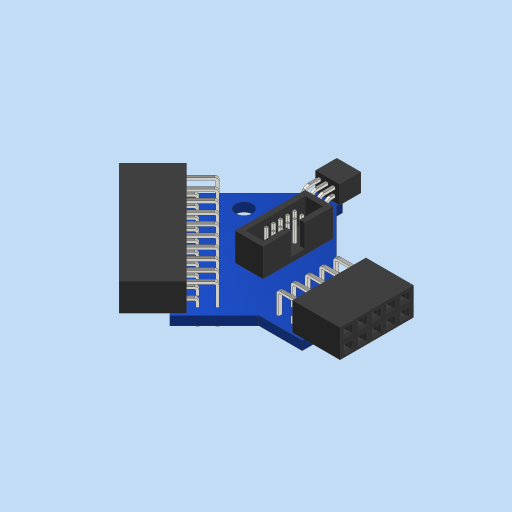
# Autodesk Inventor part: Atmel-ICE_adapter
Saved by Autodesk Inventor 2024 (Build 280153000, 153)
## iProperties
Created: 2025-05-11
Part Number: Atmel-ICE_adapter
Material: Generic
Document SubType Name: Modeling
Designer: XxPan
Density: 1 g/cm^3
Appearance: Default
Author: XxPan
Autodesk Inventor part; units mm, degrees
sketch "Sketch1" plane through (0, 0, 0) normal (0, 1, 0) x (-1, 0, 0)
  line L0 (0, 0) -> (0, -13.9)
  line L1 (0, -13.9) -> (7.7796, -13.9)
  line L2 (7.7796, -13.9) -> (17.78, -23.9005)
  line L3 (17.78, -23.9005) -> (17.78, -25.03)
  line L4 (17.78, -25.03) -> (21.78, -25.03)
  line L5 (21.78, -25.03) -> (21.78, -23.9005)
  line L6 (21.78, -23.9005) -> (34.7, -10.9805)
  line L7 (34.7, -10.9805) -> (26.2854, -2.5659)
  line L8 (26.2854, -2.5659) -> (30.8109, 1.9595)
  line L9 (30.8109, 1.9595) -> (28.6896, 4.0809)
  line L10 (28.6896, 4.0809) -> (24.1641, -0.4446)
  line L11 (24.1641, -0.4446) -> (15.7495, 7.97)
  line L12 (15.7495, 7.97) -> (7.7796, 0)
  line L13 (7.7796, 0) -> (0, 0)
  dimension "d0" = 135
  dimension "d1" = 135
  dimension "d2" = 21.1
  dimension "d3" = 13.9
  dimension "d4" = 26.8
  dimension "d5" = 11.9
  dimension "d7" = 11.9
  dimension "d8" = 6.4
  dimension "d9" = 33
  dimension "d10" = 34.7
  dimension "d11" = 4
  constraints: 28 end point, 8 perpendicular, 2 point on line, 1 horizontal alignment, 1 parallel, 1 vertical, 1 vertical alignment
  measures "d0" angle of L1 L2
  measures "d1" angle of L5 L6
  measures "d2" distance between parallel lines of L2 L7
  measures "d3" distance between parallel lines of L1 L13
  measures "d4" distance between parallel lines of L12 L6
  measures "d5" distance between parallel lines of L6 L8
  measures "d7" distance between parallel lines of L10 L12
  measures "d8" distance between parallel lines of L7 L9
  measures "d9" distance from line of L4 L11.end
  measures "d10" distance from line of L6.end L0
  measures "d11" distance of L3.end L4.end
extrude "Extrusion1" add sketch "Sketch1" against normal blind 1.6
sketch "Sketch2" plane through (0, 0, 0) normal (0, 1, 0) x (1, 0, 0)
  line L0 (-2.1, 0.375) -> (6.4, 0.375)
  line L1 (6.4, 0.375) -> (6.4, 13.525)
  line L2 (6.4, 13.525) -> (-2.1, 13.525)
  line L3 (-2.1, 13.525) -> (-2.1, 0.375)
  line L4 (-14.5828, -6.1668) -> (-20.5932, -12.1772)
  line L5 (-7.7796, 0) -> (-15.7495, -7.97) construction
  line L6 (-20.5932, -12.1772) -> (-38.9073, 6.1368)
  line L7 (-38.9073, 6.1368) -> (-32.8969, 12.1472)
  line L8 (-32.8969, 12.1472) -> (-14.5828, -6.1668)
  line L9 (-21.93, 24.33) -> (-17.63, 24.33)
  line L10 (-17.63, 24.33) -> (-17.63, 28.13)
  line L11 (-17.63, 28.13) -> (-21.93, 28.13)
  line L12 (-21.93, 28.13) -> (-21.93, 24.33)
  line L13 (-21.78, 23.9005) -> (-34.7, 10.9805) construction
  line L14 (0, 13.9) -> (-7.7796, 13.9) construction
  line L15 (-7.7796, 0) -> (0, 0) construction
  line L16 (-21.78, 25.03) -> (-21.78, 23.9005) construction
  line L17 (-17.78, 23.9005) -> (-17.78, 25.03) construction
  line L18 (0, 0) -> (0, 13.9) construction
  line L19 (-17.78, 25.03) -> (-21.78, 25.03) construction
  line L20 (-30.8109, -1.9595) -> (-28.6896, -4.0809) projected
  dimension "d14" = 4.3
  dimension "d15" = 25.9
  dimension "d16" = 8.5
  dimension "d17" = 8.5
  dimension "d18" = 13.15
  dimension "d19" = 3.8
  dimension "d20" = 26.8
  dimension "d21" = 0.45
  dimension "d22" = 13.9
  dimension "d23" = 0.375
  dimension "d24" = 4
  dimension "d25" = 0.15
  dimension "d26" = 6.4
  dimension "d27" = 3.1
  constraints: 24 end point, 7 perpendicular, 3 parallel, 2 horizontal, 1 collinear
  measures "d14" distance of L10.end L11.end
  measures "d15" distance of L4.end L6.end
  measures "d16" distance of L6.end L7.end
  measures "d17" distance of L1.end L2.end
  measures "d18" distance of L0.end L1.end
  measures "d19" distance of L11.end L9.start
  measures "d20" distance between parallel lines of L13 L5
  measures "d21" distance between parallel lines of L5 L4
  measures "d22" distance between parallel lines of L14 L15
  measures "d23" distance between parallel lines of L15 L0
  measures "d24" distance between parallel lines of L17 L16
  measures "d25" distance between parallel lines of L16 L12
  measures "d26" distance between parallel lines of L1 L18
  measures "d27" distance between parallel lines of L11 L19
extrude "Extrusion2" add sketch "Sketch2" along normal blind 5 contours L3 L2 L1 L0 | L4 L6 L7 L8
extrude "Extrusion3" add sketch "Sketch2" along normal blind 3.25 contours L12 L11 L10 L9
split_face "Split1"
sketch "Sketch3" plane through (0, 0, 0) normal (0, 1, 0) x (1, 0, 0)
  line L0 (-18.05, 6.03) -> (-13.05, 6.03)
  line L1 (-13.05, 6.03) -> (-13.05, 18.58)
  line L2 (-13.05, 18.58) -> (-18.05, 18.58)
  line L3 (-18.05, 18.58) -> (-18.05, 6.03)
  line L4 (-21.93, 24.33) -> (-17.63, 24.33) projected
  line L5 (-2.1, 13.525) -> (-2.1, 0.375) projected
  point P0 (0, 0)
  dimension "d32" = 5
  dimension "d33" = 12.55
  dimension "d34" = 5.75
  dimension "d35" = 10.95
  constraints: 8 end point, 2 parallel, 1 horizontal, 1 perpendicular
  measures "d32" distance of L1.end L2.end
  measures "d33" distance of L2.end L0.start
  measures "d34" distance between parallel lines of L4 L2
  measures "d35" distance between parallel lines of L1 L5
extrude "Extrusion4" add sketch "Sketch3" along normal blind 5 separate body
shell "Shell1" thickness 0.9 removed faces 1 at (-16.3833, 5, -14.3967) bodies 2
sketch "Sketch4" plane through (-13.05, 0, -6.03) normal (1, 0, 0) x (0, 0, -1)
  line L0 (11.65, 0.9) -> (0.9, 0.9) projected
  line L1 (0, 5) -> (12.55, 5) projected
  line L2 (11.65, 5) -> (0.9, 5) projected
  line L3 (5.05, 5) -> (5.05, 0.9)
  line L4 (7.5, 5) -> (7.5, 0.9)
  line L5 (0, 0) -> (0, 5) projected
  point P0 (-6.03, 0)
  point P1 (5.05, 5)
  dimension "d39" = 2.45
  dimension "d40" = 12.55
  dimension "d41" = 5.05
  constraints: 4 end point, 4 point on line, 2 perpendicular
  measures "d39" distance between parallel lines of L4 L3
  measures "d40" distance of L1.start L1.end
  measures "d41" distance between parallel lines of L3 L5
extrude "Extrusion5" cut sketch "Sketch4" against normal up to surface (0.9 mm away) bodies 2
sketch "Sketch5" plane through (0, 0, 0) normal (0, 1, 0) x (1, 0, 0)
  circle A0 centre (-25.649, 15.2231) radius 1.5
  line L0 (-34.3818, 10.6623) -> (-26.2854, 2.5659) projected
  line L1 (-21.78, 23.9005) -> (-34.7, 10.9805) projected
  point P0 (0, 0)
  dimension "d44" = 3
  dimension "d45" = 7.9
  dimension "d46" = 1.9
  constraints: 1 centre point
  measures "d44" diameter of A0
  measures "d45" distance edge to line of A0 L0
  measures "d46" distance edge to line of A0 L1
extrude "Extrusion6" cut sketch "Sketch5" against normal through all bodies 1
sketch "Sketch6" plane through (-17.15, 0.9, -17.68) normal (0, 1, 0) x (1, 0, 0)
  line L0 (0.765, -8.115) -> (1.165, -8.115)
  line L1 (1.165, -8.115) -> (1.165, -7.715)
  line L2 (1.165, -7.715) -> (0.765, -7.715)
  line L3 (0.765, -7.715) -> (0.765, -8.115)
  line L4 (0.765, -8.115) -> (1.165, -7.715) construction
  line L5 (1.165, -8.115) -> (0.765, -7.715) construction
  line L6 (0.765, -6.845) -> (1.165, -6.845)
  line L7 (1.165, -6.845) -> (1.165, -6.445)
  line L8 (1.165, -6.445) -> (0.765, -6.445)
  line L9 (0.765, -6.445) -> (0.765, -6.845)
  line L10 (0.765, -6.845) -> (1.165, -6.445) construction
  line L11 (1.165, -6.845) -> (0.765, -6.445) construction
  line L12 (0.765, -5.575) -> (1.165, -5.575)
  line L13 (1.165, -5.575) -> (1.165, -5.175)
  line L14 (1.165, -5.175) -> (0.765, -5.175)
  line L15 (0.765, -5.175) -> (0.765, -5.575)
  line L16 (0.765, -5.575) -> (1.165, -5.175) construction
  line L17 (1.165, -5.575) -> (0.765, -5.175) construction
  line L18 (0.765, -4.305) -> (1.165, -4.305)
  line L19 (1.165, -4.305) -> (1.165, -3.905)
  line L20 (1.165, -3.905) -> (0.765, -3.905)
  line L21 (0.765, -3.905) -> (0.765, -4.305)
  line L22 (0.765, -4.305) -> (1.165, -3.905) construction
  line L23 (1.165, -4.305) -> (0.765, -3.905) construction
  line L24 (0.765, -3.035) -> (1.165, -3.035)
  line L25 (1.165, -3.035) -> (1.165, -2.635)
  line L26 (1.165, -2.635) -> (0.765, -2.635)
  line L27 (0.765, -2.635) -> (0.765, -3.035)
  line L28 (0.765, -3.035) -> (1.165, -2.635) construction
  line L29 (1.165, -3.035) -> (0.765, -2.635) construction
  line L30 (2.035, -8.115) -> (2.435, -8.115)
  line L31 (2.435, -8.115) -> (2.435, -7.715)
  line L32 (2.435, -7.715) -> (2.035, -7.715)
  line L33 (2.035, -7.715) -> (2.035, -8.115)
  line L34 (2.035, -8.115) -> (2.435, -7.715) construction
  line L35 (2.435, -8.115) -> (2.035, -7.715) construction
  line L36 (2.035, -6.845) -> (2.435, -6.845)
  line L37 (2.435, -6.845) -> (2.435, -6.445)
  line L38 (2.435, -6.445) -> (2.035, -6.445)
  line L39 (2.035, -6.445) -> (2.035, -6.845)
  line L40 (2.035, -6.845) -> (2.435, -6.445) construction
  line L41 (2.435, -6.845) -> (2.035, -6.445) construction
  line L42 (2.035, -5.575) -> (2.435, -5.575)
  line L43 (2.435, -5.575) -> (2.435, -5.175)
  line L44 (2.435, -5.175) -> (2.035, -5.175)
  line L45 (2.035, -5.175) -> (2.035, -5.575)
  line L46 (2.035, -5.575) -> (2.435, -5.175) construction
  line L47 (2.435, -5.575) -> (2.035, -5.175) construction
  line L48 (2.035, -4.305) -> (2.435, -4.305)
  line L49 (2.435, -4.305) -> (2.435, -3.905)
  line L50 (2.435, -3.905) -> (2.035, -3.905)
  line L51 (2.035, -3.905) -> (2.035, -4.305)
  line L52 (2.035, -4.305) -> (2.435, -3.905) construction
  line L53 (2.435, -4.305) -> (2.035, -3.905) construction
  line L54 (2.035, -3.035) -> (2.435, -3.035)
  line L55 (2.435, -3.035) -> (2.435, -2.635)
  line L56 (2.435, -2.635) -> (2.035, -2.635)
  line L57 (2.035, -2.635) -> (2.035, -3.035)
  line L58 (2.035, -3.035) -> (2.435, -2.635) construction
  line L59 (2.435, -3.035) -> (2.035, -2.635) construction
  line L60 (3.2, -10.75) -> (0, -10.75) projected
  line L61 (0, 0) -> (3.2, 0) projected
  line L62 (0, -10.75) -> (0, 0) projected
  line L63 (3.2, 0) -> (3.2, -4.15) projected
  line L64 (0.965, -7.915) -> (2.235, -7.915) construction
  point P0 (17.15, -17.68)
  point P1 (0.965, -6.645)
  point P2 (0.965, -5.375)
  point P3 (0.965, -4.105)
  point P4 (0.965, -2.835)
  point P5 (2.235, -6.645)
  point P6 (2.235, -5.375)
  point P7 (2.235, -4.105)
  point P8 (2.235, -2.835)
  point P9 (1.6, -7.915)
  point P10 (1.6, -10.75)
  point P11 (0.965, -5.375)
  point P12 (0, -5.375)
  dimension "d49" = 0.4
  dimension "d50" = 0.4
  dimension "d53" = 1.27
  dimension "d56" = 1.27
  constraints: 122 end point, 6 midpoint, 3 horizontal, 2 collinear, 2 parallel, 1 horizontal alignment, 1 perpendicular, 1 vertical, 1 vertical alignment, 97 other
  measures "d49" distance of L2.end L1.end
  measures "d50" distance of L1.end L0.end
  measures "d53" distance of L0.start L6.start
  measures "d56" distance of L0.start L30.start
extrude "Extrusion7" add sketch "Sketch6" along normal blind 3.75 and the other way blind 3 bodies 2
ref_plane "Work Plane1" through (-15.4808, 0, 5.2688) normal (0.7071068, 0, 0.7071068) x (0.7071068, 0, -0.7071068)
sketch "Sketch7" plane through (-15.4808, 0, 5.2688) normal (0.7071068, 0, 0.7071068) x (0.7071068, 0, -0.7071068)
  line L0 (0, 0) -> (0, 5) construction
  line L1 (0, 3.97) -> (3.55, 3.97)
  line L2 (4.15, 3.37) -> (4.15, -2.93)
  line L3 (4.15, -2.93) -> (3.75, -2.93)
  line L4 (3.75, -2.93) -> (3.75, 3.37)
  line L5 (3.55, 3.57) -> (0, 3.57)
  line L6 (0, 1.43) -> (1.01, 1.43)
  line L7 (1.61, 0.83) -> (1.61, -2.93)
  line L8 (1.61, -2.93) -> (1.21, -2.93)
  line L9 (1.21, -2.93) -> (1.21, 0.83)
  line L10 (1.01, 1.03) -> (0, 1.03)
  line L11 (0, 3.97) -> (0, 3.57)
  line L12 (0, 1.43) -> (0, 1.03)
  arc A0 (1.21, 0.83) -> (1.01, 1.03) centre (1.01, 0.83) ccw
  arc A1 (3.75, 3.37) -> (3.55, 3.57) centre (3.55, 3.37) ccw
  arc A2 (1.61, 0.83) -> (1.01, 1.43) centre (1.01, 0.83) ccw
  arc A3 (4.15, 3.37) -> (3.55, 3.97) centre (3.55, 3.37) ccw
  line L13 (0, 3.77) -> (0, 5)
  line L14 (0, 1.23) -> (0, 0)
  line L15 (-8.5, 0) -> (-8.5, 5) projected
  point P0 (14.6722, 0)
  point P1 (3.95, -2.93)
  point P2 (1.41, -2.93)
  dimension "d62" = 2.54
  dimension "d63" = 2.54
  dimension "d64" = 0.4
  dimension "d66" = 0.2
  dimension "d67" = 0.6
  dimension "d68" = 12.65
  dimension "d69" = 6.9
  constraints: 28 end point, 8 point on circle, 8 tangent, 7 perpendicular, 6 point on line, 4 centre point, 4 collinear, 4 equal length, 4 midpoint, 2 equal radius, 1 horizontal, 1 parallel
  measures "d62" distance of L14.start L13.start
  measures "d63" distance of point (3.95, -2.93) point (1.41, -2.93)
  measures "d64" distance of L2.end L3.end
  measures "d66" radius of A0
  measures "d67" radius of A2
  measures "d68" distance between parallel lines of L15 L2
  measures "d69" distance between parallel lines of L8 L1
extrude "Extrusion8" add sketch "Sketch7" against normal blind 0.6 bodies 1
pattern_linear "Rectangular Pattern1" count 10 spacing 2.54 along (-0.7071068, 0, -0.7071068) of "Extrusion8" bodies 1
ref_plane "Work Plane2" through (0, 0, -1.645) normal (0, 0, 1) x (1, 0, 0)
sketch "Sketch8" plane through (0, 0, -1.645) normal (0, 0, 1) x (1, 0, 0)
  line L0 (-2.1, 0) -> (-2.1, 5) projected
  line L1 (-2.1, 3.97) -> (-2.1, 3.57)
  line L2 (-2.1, 3.57) -> (-5.65, 3.57)
  line L3 (-5.85, 3.37) -> (-5.85, -3.03)
  line L4 (-5.85, -3.03) -> (-6.25, -3.03)
  line L5 (-6.25, -3.03) -> (-6.25, 3.37)
  line L6 (-5.65, 3.97) -> (-2.1, 3.97)
  line L7 (-2.1, 1.43) -> (-2.1, 1.03)
  line L8 (-2.1, 1.03) -> (-3.11, 1.03)
  line L9 (-3.31, 0.83) -> (-3.31, -3.03)
  line L10 (-3.31, -3.03) -> (-3.71, -3.03)
  line L11 (-3.71, -3.03) -> (-3.71, 0.83)
  line L12 (-3.11, 1.43) -> (-2.1, 1.43)
  line L13 (-2.1, 1.23) -> (-2.1, 0)
  line L14 (-2.1, 3.77) -> (-2.1, 5)
  line L15 (6.4, 0) -> (6.4, 5) projected
  arc A0 (-5.65, 3.57) -> (-5.85, 3.37) centre (-5.65, 3.37) ccw
  arc A1 (-3.11, 1.03) -> (-3.31, 0.83) centre (-3.11, 0.83) ccw
  arc A2 (-3.11, 1.43) -> (-3.71, 0.83) centre (-3.11, 0.83) ccw
  arc A3 (-5.65, 3.97) -> (-6.25, 3.37) centre (-5.65, 3.37) ccw
  point P0 (0, 0)
  point P1 (-6.05, -3.03)
  point P2 (-3.51, -3.03)
  dimension "d76" = 0.4
  dimension "d77" = 0.4
  dimension "d78" = 0.4
  dimension "d79" = 0.4
  dimension "d80" = 2.54
  dimension "d81" = 2.54
  dimension "d82" = 12.65
  dimension "d83" = 7
  dimension "d84" = 0.2
  dimension "d85" = 0.6
  constraints: 28 end point, 9 perpendicular, 8 point on circle, 8 tangent, 4 centre point, 4 collinear, 4 midpoint, 4 point on line, 2 equal radius, 1 vertical
  measures "d76" distance of L1.start L1.end
  measures "d77" distance of L3.end L4.end
  measures "d78" distance of L7.start L7.end
  measures "d79" distance of L9.end L10.end
  measures "d80" distance of L13.start L14.start
  measures "d81" distance of point (-6.05, -3.03) point (-3.51, -3.03)
  measures "d82" distance between parallel lines of L15 L5
  measures "d83" distance between parallel lines of L4 L6
  measures "d84" radius of A0
  measures "d85" radius of A2
extrude "Extrusion9" add sketch "Sketch8" against normal blind 0.6 bodies 1
pattern_linear "Rectangular Pattern2" count 5 spacing 2.54 along (0, 0, -1) of "Extrusion9" bodies 1
ref_plane "Work Plane3" through (-18.43, 0, -24.33) normal (1, 0, 0) x (0, 0, -1)
sketch "Sketch9" plane through (-18.43, 0, -24.33) normal (1, 0, 0) x (0, 0, -1)
  line L0 (0, 0) -> (0, 3.25) projected
  line L1 (0, 2.485) -> (0, 2.035)
  line L2 (0, 2.035) -> (-1.85, 2.035)
  line L3 (-2.65, 1.235) -> (-2.65, -2.815)
  line L4 (-2.65, -2.815) -> (-3.1, -2.815)
  line L5 (-3.1, -2.815) -> (-3.1, 1.235)
  line L6 (-1.85, 2.485) -> (0, 2.485)
  line L7 (0, 1.215) -> (0, 0.765)
  line L8 (0, 0.765) -> (-0.58, 0.765)
  line L9 (-1.38, -0.035) -> (-1.38, -2.815)
  line L10 (-1.38, -2.815) -> (-1.83, -2.815)
  line L11 (-1.83, -2.815) -> (-1.83, -0.035)
  line L12 (-0.58, 1.215) -> (0, 1.215)
  line L13 (0, 2.26) -> (0, 3.25)
  line L14 (0, 0.99) -> (0, 0)
  line L15 (3.8, 0) -> (3.8, 3.25) projected
  arc A0 (-0.58, 0.765) -> (-1.38, -0.035) centre (-0.58, -0.035) ccw
  arc A1 (-1.85, 2.035) -> (-2.65, 1.235) centre (-1.85, 1.235) ccw
  arc A2 (-1.85, 2.485) -> (-3.1, 1.235) centre (-1.85, 1.235) ccw
  arc A3 (-0.58, 1.215) -> (-1.83, -0.035) centre (-0.58, -0.035) ccw
  point P0 (-24.33, 0)
  point P1 (-2.875, -2.815)
  point P2 (-1.605, -2.815)
  point P3 (0, 0.765)
  point P4 (0, 1.215)
  dimension "d92" = 0.45
  dimension "d93" = 0.45
  dimension "d94" = 0.45
  dimension "d95" = 0.45
  dimension "d96" = 1.27
  dimension "d97" = 1.27
  dimension "d98" = 6.9
  dimension "d99" = 5.3
  dimension "d100" = 0.8
  dimension "d101" = 1.25
  constraints: 28 end point, 9 perpendicular, 8 point on circle, 8 tangent, 6 point on line, 4 centre point, 4 midpoint, 3 collinear, 2 equal radius
  measures "d92" distance of L1.start L1.end
  measures "d93" distance of L3.end L4.end
  measures "d94" distance of L7.start L7.end
  measures "d95" distance of L9.end L10.end
  measures "d96" distance of L13.start L14.start
  measures "d97" distance of point (-2.875, -2.815) point (-1.605, -2.815)
  measures "d98" distance between parallel lines of L15 L5
  measures "d99" distance between parallel lines of L6 L10
  measures "d100" radius of A0
  measures "d101" radius of A2
extrude "Extrusion10" add sketch "Sketch9" against normal blind 0.45 bodies 1
pattern_linear "Rectangular Pattern3" count 3 spacing 1.27 along (-1, 0, 0) of "Extrusion10" bodies 1
sketch "Sketch10" plane through (-20.5932, 0, 12.1772) normal (-0.7071068, 0, 0.7071068) x (0.7071068, 0, 0.7071068)
  line L0 (-24.8, 4.13) -> (-24, 4.13)
  line L1 (-24, 4.13) -> (-24, 3.33)
  line L2 (-24, 3.33) -> (-24.8, 3.33)
  line L3 (-24.8, 3.33) -> (-24.8, 4.13)
  line L4 (-24.8, 4.13) -> (-24, 3.33) construction
  line L5 (-24, 4.13) -> (-24.8, 3.33) construction
  line L6 (-22.26, 4.13) -> (-21.46, 4.13)
  line L7 (-21.46, 4.13) -> (-21.46, 3.33)
  line L8 (-21.46, 3.33) -> (-22.26, 3.33)
  line L9 (-22.26, 3.33) -> (-22.26, 4.13)
  line L10 (-22.26, 4.13) -> (-21.46, 3.33) construction
  line L11 (-21.46, 4.13) -> (-22.26, 3.33) construction
  line L12 (-19.72, 4.13) -> (-18.92, 4.13)
  line L13 (-18.92, 4.13) -> (-18.92, 3.33)
  line L14 (-18.92, 3.33) -> (-19.72, 3.33)
  line L15 (-19.72, 3.33) -> (-19.72, 4.13)
  line L16 (-19.72, 4.13) -> (-18.92, 3.33) construction
  line L17 (-18.92, 4.13) -> (-19.72, 3.33) construction
  line L18 (-17.18, 4.13) -> (-16.38, 4.13)
  line L19 (-16.38, 4.13) -> (-16.38, 3.33)
  line L20 (-16.38, 3.33) -> (-17.18, 3.33)
  line L21 (-17.18, 3.33) -> (-17.18, 4.13)
  line L22 (-17.18, 4.13) -> (-16.38, 3.33) construction
  line L23 (-16.38, 4.13) -> (-17.18, 3.33) construction
  line L24 (-14.64, 4.13) -> (-13.84, 4.13)
  line L25 (-13.84, 4.13) -> (-13.84, 3.33)
  line L26 (-13.84, 3.33) -> (-14.64, 3.33)
  line L27 (-14.64, 3.33) -> (-14.64, 4.13)
  line L28 (-14.64, 4.13) -> (-13.84, 3.33) construction
  line L29 (-13.84, 4.13) -> (-14.64, 3.33) construction
  line L30 (-12.1, 4.13) -> (-11.3, 4.13)
  line L31 (-11.3, 4.13) -> (-11.3, 3.33)
  line L32 (-11.3, 3.33) -> (-12.1, 3.33)
  line L33 (-12.1, 3.33) -> (-12.1, 4.13)
  line L34 (-12.1, 4.13) -> (-11.3, 3.33) construction
  line L35 (-11.3, 4.13) -> (-12.1, 3.33) construction
  line L36 (-9.56, 4.13) -> (-8.76, 4.13)
  line L37 (-8.76, 4.13) -> (-8.76, 3.33)
  line L38 (-8.76, 3.33) -> (-9.56, 3.33)
  line L39 (-9.56, 3.33) -> (-9.56, 4.13)
  line L40 (-9.56, 4.13) -> (-8.76, 3.33) construction
  line L41 (-8.76, 4.13) -> (-9.56, 3.33) construction
  line L42 (-7.02, 4.13) -> (-6.22, 4.13)
  line L43 (-6.22, 4.13) -> (-6.22, 3.33)
  line L44 (-6.22, 3.33) -> (-7.02, 3.33)
  line L45 (-7.02, 3.33) -> (-7.02, 4.13)
  line L46 (-7.02, 4.13) -> (-6.22, 3.33) construction
  line L47 (-6.22, 4.13) -> (-7.02, 3.33) construction
  line L48 (-4.48, 4.13) -> (-3.68, 4.13)
  line L49 (-3.68, 4.13) -> (-3.68, 3.33)
  line L50 (-3.68, 3.33) -> (-4.48, 3.33)
  line L51 (-4.48, 3.33) -> (-4.48, 4.13)
  line L52 (-4.48, 4.13) -> (-3.68, 3.33) construction
  line L53 (-3.68, 4.13) -> (-4.48, 3.33) construction
  line L54 (-1.94, 4.13) -> (-1.14, 4.13)
  line L55 (-1.14, 4.13) -> (-1.14, 3.33)
  line L56 (-1.14, 3.33) -> (-1.94, 3.33)
  line L57 (-1.94, 3.33) -> (-1.94, 4.13)
  line L58 (-1.94, 4.13) -> (-1.14, 3.33) construction
  line L59 (-1.14, 4.13) -> (-1.94, 3.33) construction
  line L60 (-24.8, 1.59) -> (-24, 1.59)
  line L61 (-24, 1.59) -> (-24, 0.79)
  line L62 (-24, 0.79) -> (-24.8, 0.79)
  line L63 (-24.8, 0.79) -> (-24.8, 1.59)
  line L64 (-24.8, 1.59) -> (-24, 0.79) construction
  line L65 (-24, 1.59) -> (-24.8, 0.79) construction
  line L66 (-22.26, 1.59) -> (-21.46, 1.59)
  line L67 (-21.46, 1.59) -> (-21.46, 0.79)
  line L68 (-21.46, 0.79) -> (-22.26, 0.79)
  line L69 (-22.26, 0.79) -> (-22.26, 1.59)
  line L70 (-22.26, 1.59) -> (-21.46, 0.79) construction
  line L71 (-21.46, 1.59) -> (-22.26, 0.79) construction
  line L72 (-19.72, 1.59) -> (-18.92, 1.59)
  line L73 (-18.92, 1.59) -> (-18.92, 0.79)
  line L74 (-18.92, 0.79) -> (-19.72, 0.79)
  line L75 (-19.72, 0.79) -> (-19.72, 1.59)
  line L76 (-19.72, 1.59) -> (-18.92, 0.79) construction
  line L77 (-18.92, 1.59) -> (-19.72, 0.79) construction
  line L78 (-17.18, 1.59) -> (-16.38, 1.59)
  line L79 (-16.38, 1.59) -> (-16.38, 0.79)
  line L80 (-16.38, 0.79) -> (-17.18, 0.79)
  line L81 (-17.18, 0.79) -> (-17.18, 1.59)
  line L82 (-17.18, 1.59) -> (-16.38, 0.79) construction
  line L83 (-16.38, 1.59) -> (-17.18, 0.79) construction
  line L84 (-14.64, 1.59) -> (-13.84, 1.59)
  line L85 (-13.84, 1.59) -> (-13.84, 0.79)
  line L86 (-13.84, 0.79) -> (-14.64, 0.79)
  line L87 (-14.64, 0.79) -> (-14.64, 1.59)
  line L88 (-14.64, 1.59) -> (-13.84, 0.79) construction
  line L89 (-13.84, 1.59) -> (-14.64, 0.79) construction
  line L90 (-12.1, 1.59) -> (-11.3, 1.59)
  line L91 (-11.3, 1.59) -> (-11.3, 0.79)
  line L92 (-11.3, 0.79) -> (-12.1, 0.79)
  line L93 (-12.1, 0.79) -> (-12.1, 1.59)
  line L94 (-12.1, 1.59) -> (-11.3, 0.79) construction
  line L95 (-11.3, 1.59) -> (-12.1, 0.79) construction
  line L96 (-9.56, 1.59) -> (-8.76, 1.59)
  line L97 (-8.76, 1.59) -> (-8.76, 0.79)
  line L98 (-8.76, 0.79) -> (-9.56, 0.79)
  line L99 (-9.56, 0.79) -> (-9.56, 1.59)
  line L100 (-9.56, 1.59) -> (-8.76, 0.79) construction
  line L101 (-8.76, 1.59) -> (-9.56, 0.79) construction
  line L102 (-7.02, 1.59) -> (-6.22, 1.59)
  line L103 (-6.22, 1.59) -> (-6.22, 0.79)
  line L104 (-6.22, 0.79) -> (-7.02, 0.79)
  line L105 (-7.02, 0.79) -> (-7.02, 1.59)
  line L106 (-7.02, 1.59) -> (-6.22, 0.79) construction
  line L107 (-6.22, 1.59) -> (-7.02, 0.79) construction
  line L108 (-4.48, 1.59) -> (-3.68, 1.59)
  line L109 (-3.68, 1.59) -> (-3.68, 0.79)
  line L110 (-3.68, 0.79) -> (-4.48, 0.79)
  line L111 (-4.48, 0.79) -> (-4.48, 1.59)
  line L112 (-4.48, 1.59) -> (-3.68, 0.79) construction
  line L113 (-3.68, 1.59) -> (-4.48, 0.79) construction
  line L114 (-1.94, 1.59) -> (-1.14, 1.59)
  line L115 (-1.14, 1.59) -> (-1.14, 0.79)
  line L116 (-1.14, 0.79) -> (-1.94, 0.79)
  line L117 (-1.94, 0.79) -> (-1.94, 1.59)
  line L118 (-1.94, 1.59) -> (-1.14, 0.79) construction
  line L119 (-1.14, 1.59) -> (-1.94, 0.79) construction
  line L120 (-25.9, 5) -> (0, 5) projected
  line L121 (-25.9, 0) -> (-25.9, 5) projected
  point P0 (5.951, 0)
  point P1 (-24.4, 3.73)
  point P2 (-21.86, 3.73)
  point P3 (-19.32, 3.73)
  point P4 (-16.78, 3.73)
  point P5 (-14.24, 3.73)
  point P6 (-11.7, 3.73)
  point P7 (-9.16, 3.73)
  point P8 (-6.62, 3.73)
  point P9 (-4.08, 3.73)
  point P10 (-1.54, 3.73)
  point P11 (-24.4, 1.19)
  point P12 (-21.86, 1.19)
  point P13 (-19.32, 1.19)
  point P14 (-16.78, 1.19)
  point P15 (-14.24, 1.19)
  point P16 (-11.7, 1.19)
  point P17 (-9.16, 1.19)
  point P18 (-6.62, 1.19)
  point P19 (-4.08, 1.19)
  point P20 (-1.54, 1.19)
  dimension "d109" = 0.8
  dimension "d110" = 0.8
  dimension "d113" = 2.54
  dimension "d116" = 2.54
  dimension "d119" = 1.27
  dimension "d120" = 1.5
  constraints: 240 end point, 2 collinear, 2 horizontal, 2 midpoint, 2 parallel, 1 perpendicular, 1 vertical, 207 other
  measures "d109" distance of L1.end L2.end
  measures "d110" distance of L0.end L1.end
  measures "d113" distance of L0.start L6.start
  measures "d116" distance of L0.start L60.start
  measures "d119" distance from line of L120 point (-24.4, 3.73)
  measures "d120" distance from line of L121 point (-24.4, 3.73)
extrude "Extrusion11" cut sketch "Sketch10" against normal blind 6 bodies 1
chamfer "Chamfer1" distance 0.4 angle 45 80 edges at (-37.8466, 3.33, -5.0762) (-38.1295, 3.73, -5.359) (-37.8466, 4.13, -5.0762) (-37.5638, 3.73, -4.7933) (-37.8466, 1.59, -5.0762) (-38.1295, 1.19, -5.359) (-37.8466, 0.79, -5.0762) (-37.5638, 1.19, -4.7933) (-36.3334, 3.73, -3.563) (-36.0506, 4.13, -3.2801) (-35.7677, 3.73, -2.9973) (-36.0506, 3.33, -3.2801) (-36.0506, 1.59, -3.2801) (-36.3334, 1.19, -3.563) (-36.0506, 0.79, -3.2801) (-35.7677, 1.19, -2.9973) (-34.5374, 1.19, -1.7669) (-34.2545, 1.59, -1.4841) (-33.9717, 1.19, -1.2012) (-34.2545, 0.79, -1.4841) (-34.2545, 3.33, -1.4841) (-34.5374, 3.73, -1.7669) (-34.2545, 4.13, -1.4841) (-33.9717, 3.73, -1.2012) (-32.7413, 3.73, 0.0291) (-32.4585, 3.33, 0.312) (-32.1756, 3.73, 0.5948) (-32.4585, 4.13, 0.312) (-32.4585, 1.59, 0.312) (-32.7413, 1.19, 0.0291) (-32.4585, 0.79, 0.312) (-32.1756, 1.19, 0.5948) (-30.9453, 1.19, 1.8252) (-30.6624, 0.79, 2.108) (-30.6624, 1.59, 2.108) (-30.3796, 1.19, 2.3909) (-30.6624, 3.33, 2.108) (-30.9453, 3.73, 1.8252) (-30.6624, 4.13, 2.108) (-30.3796, 3.73, 2.3909) (-28.8664, 4.13, 3.9041) (-29.1492, 3.73, 3.6212) (-28.8664, 3.33, 3.9041) (-28.5835, 3.73, 4.1869) (-28.8664, 1.59, 3.9041) (-29.1492, 1.19, 3.6212) (-28.8664, 0.79, 3.9041) (-28.5835, 1.19, 4.1869) (-27.3532, 1.19, 5.4173) (-27.0703, 0.79, 5.7001) (-27.0703, 1.59, 5.7001) (-26.7875, 1.19, 5.983) (-26.7875, 3.73, 5.983) (-27.0703, 3.33, 5.7001) (-27.3532, 3.73, 5.4173) (-27.0703, 4.13, 5.7001) (-25.2743, 1.59, 7.4962) (-25.5571, 1.19, 7.2133) (-25.2743, 0.79, 7.4962) (-24.9914, 1.19, 7.779) (-25.2743, 3.33, 7.4962) (-25.2743, 4.13, 7.4962) (-25.5571, 3.73, 7.2133) (-24.9914, 3.73, 7.779) (-23.7611, 3.73, 9.0094) (-23.4782, 4.13, 9.2922) (-23.1954, 3.73, 9.5751) (-23.4782, 3.33, 9.2922) (-23.4782, 1.59, 9.2922) (-23.7611, 1.19, 9.0094) (-23.4782, 0.79, 9.2922) (-23.1954, 1.19, 9.5751) (-21.965, 1.19, 10.8055) (-21.6822, 0.79, 11.0883) (-21.3993, 1.19, 11.3711) (-21.6822, 1.59, 11.0883) (-21.6822, 3.33, 11.0883) (-21.965, 3.73, 10.8055) (-21.6822, 4.13, 11.0883) (-21.3993, 3.73, 11.3711)
sketch "Sketch11" plane through (6.4, 0, -0.375) normal (1, 0, 0) x (0, 0, -1)
  line L0 (1.1, 4.13) -> (1.9, 4.13)
  line L1 (1.9, 4.13) -> (1.9, 3.33)
  line L2 (1.9, 3.33) -> (1.1, 3.33)
  line L3 (1.1, 3.33) -> (1.1, 4.13)
  line L4 (1.1, 4.13) -> (1.9, 3.33) construction
  line L5 (1.9, 4.13) -> (1.1, 3.33) construction
  line L6 (3.64, 4.13) -> (4.44, 4.13)
  line L7 (4.44, 4.13) -> (4.44, 3.33)
  line L8 (4.44, 3.33) -> (3.64, 3.33)
  line L9 (3.64, 3.33) -> (3.64, 4.13)
  line L10 (3.64, 4.13) -> (4.44, 3.33) construction
  line L11 (4.44, 4.13) -> (3.64, 3.33) construction
  line L12 (6.18, 4.13) -> (6.98, 4.13)
  line L13 (6.98, 4.13) -> (6.98, 3.33)
  line L14 (6.98, 3.33) -> (6.18, 3.33)
  line L15 (6.18, 3.33) -> (6.18, 4.13)
  line L16 (6.18, 4.13) -> (6.98, 3.33) construction
  line L17 (6.98, 4.13) -> (6.18, 3.33) construction
  line L18 (8.72, 4.13) -> (9.52, 4.13)
  line L19 (9.52, 4.13) -> (9.52, 3.33)
  line L20 (9.52, 3.33) -> (8.72, 3.33)
  line L21 (8.72, 3.33) -> (8.72, 4.13)
  line L22 (8.72, 4.13) -> (9.52, 3.33) construction
  line L23 (9.52, 4.13) -> (8.72, 3.33) construction
  line L24 (11.26, 4.13) -> (12.06, 4.13)
  line L25 (12.06, 4.13) -> (12.06, 3.33)
  line L26 (12.06, 3.33) -> (11.26, 3.33)
  line L27 (11.26, 3.33) -> (11.26, 4.13)
  line L28 (11.26, 4.13) -> (12.06, 3.33) construction
  line L29 (12.06, 4.13) -> (11.26, 3.33) construction
  line L30 (1.1, 1.59) -> (1.9, 1.59)
  line L31 (1.9, 1.59) -> (1.9, 0.79)
  line L32 (1.9, 0.79) -> (1.1, 0.79)
  line L33 (1.1, 0.79) -> (1.1, 1.59)
  line L34 (1.1, 1.59) -> (1.9, 0.79) construction
  line L35 (1.9, 1.59) -> (1.1, 0.79) construction
  line L36 (3.64, 1.59) -> (4.44, 1.59)
  line L37 (4.44, 1.59) -> (4.44, 0.79)
  line L38 (4.44, 0.79) -> (3.64, 0.79)
  line L39 (3.64, 0.79) -> (3.64, 1.59)
  line L40 (3.64, 1.59) -> (4.44, 0.79) construction
  line L41 (4.44, 1.59) -> (3.64, 0.79) construction
  line L42 (6.18, 1.59) -> (6.98, 1.59)
  line L43 (6.98, 1.59) -> (6.98, 0.79)
  line L44 (6.98, 0.79) -> (6.18, 0.79)
  line L45 (6.18, 0.79) -> (6.18, 1.59)
  line L46 (6.18, 1.59) -> (6.98, 0.79) construction
  line L47 (6.98, 1.59) -> (6.18, 0.79) construction
  line L48 (8.72, 1.59) -> (9.52, 1.59)
  line L49 (9.52, 1.59) -> (9.52, 0.79)
  line L50 (9.52, 0.79) -> (8.72, 0.79)
  line L51 (8.72, 0.79) -> (8.72, 1.59)
  line L52 (8.72, 1.59) -> (9.52, 0.79) construction
  line L53 (9.52, 1.59) -> (8.72, 0.79) construction
  line L54 (11.26, 1.59) -> (12.06, 1.59)
  line L55 (12.06, 1.59) -> (12.06, 0.79)
  line L56 (12.06, 0.79) -> (11.26, 0.79)
  line L57 (11.26, 0.79) -> (11.26, 1.59)
  line L58 (11.26, 1.59) -> (12.06, 0.79) construction
  line L59 (12.06, 1.59) -> (11.26, 0.79) construction
  line L60 (0, 0) -> (0, 5) projected
  line L61 (0, 5) -> (13.15, 5) projected
  point P0 (-0.375, 0)
  point P1 (1.5, 3.73)
  point P2 (4.04, 3.73)
  point P3 (6.58, 3.73)
  point P4 (9.12, 3.73)
  point P5 (11.66, 3.73)
  point P6 (1.5, 1.19)
  point P7 (4.04, 1.19)
  point P8 (6.58, 1.19)
  point P9 (9.12, 1.19)
  point P10 (11.66, 1.19)
  dimension "d126" = 0.8
  dimension "d127" = 0.8
  dimension "d130" = 2.54
  dimension "d133" = 2.54
  dimension "d136" = 1.5
  dimension "d137" = 1.27
  constraints: 120 end point, 2 collinear, 2 horizontal, 2 midpoint, 2 parallel, 1 perpendicular, 1 vertical, 97 other
  measures "d126" distance of L1.end L2.end
  measures "d127" distance of L0.end L1.end
  measures "d130" distance of L0.start L6.start
  measures "d133" distance of L0.start L30.start
  measures "d136" distance from line of L60 point (1.5, 3.73)
  measures "d137" distance from line of L61 point (1.5, 3.73)
extrude "Extrusion12" cut sketch "Sketch11" against normal blind 6 bodies 1
chamfer "Chamfer2" distance 0.4 angle 45 40 edges at (6.4, 4.13, -1.875) (6.4, 3.73, -1.475) (6.4, 3.33, -1.875) (6.4, 3.73, -2.275) (6.4, 1.59, -1.875) (6.4, 1.19, -1.475) (6.4, 0.79, -1.875) (6.4, 1.19, -2.275) (6.4, 1.19, -4.015) (6.4, 1.59, -4.415) (6.4, 1.19, -4.815) (6.4, 0.79, -4.415) (6.4, 1.19, -6.555) (6.4, 0.79, -6.955) (6.4, 1.59, -6.955) (6.4, 1.19, -7.355) (6.4, 3.33, -6.955) (6.4, 3.73, -6.555) (6.4, 4.13, -6.955) (6.4, 3.73, -7.355) (6.4, 3.73, -4.815) (6.4, 3.33, -4.415) (6.4, 3.73, -4.015) (6.4, 4.13, -4.415) (6.4, 4.13, -9.495) (6.4, 3.73, -9.095) (6.4, 3.33, -9.495) (6.4, 3.73, -9.895) (6.4, 4.13, -12.035) (6.4, 3.73, -11.635) (6.4, 3.33, -12.035) (6.4, 3.73, -12.435) (6.4, 1.59, -12.035) (6.4, 1.19, -11.635) (6.4, 0.79, -12.035) (6.4, 1.19, -12.435) (6.4, 1.59, -9.495) (6.4, 1.19, -9.095) (6.4, 0.79, -9.495) (6.4, 1.19, -9.895)
sketch "Sketch12" plane through (-17.63, 0, -28.13) normal (0, 0, -1) x (-1, 0, 0)
  circle A0 centre (0.9, 2.25) radius 0.25
  line L0 (0.9, 2.25) -> (1.9679, 2.25) construction
  line L1 (0.9, 2.25) -> (0.9, 6.4223) construction
  circle A1 centre (2.17, 2.25) radius 0.25
  circle A2 centre (3.44, 2.25) radius 0.25
  circle A3 centre (0.9, 0.98) radius 0.25
  circle A4 centre (2.17, 0.98) radius 0.25
  circle A5 centre (3.44, 0.98) radius 0.25
  line L2 (0, 0) -> (0, 3.25) projected
  line L3 (0, 3.25) -> (4.3, 3.25) projected
  point P0 (-17.63, 0)
  dimension "d143" = 0.5
  dimension "d146" = 1.27
  dimension "d149" = 1.27
  dimension "d152" = 0.9
  dimension "d153" = 1
  constraints: 6 centre point, 4 end point, 2 horizontal, 2 vertical, 10 other
  measures "d143" diameter of A0
  measures "d146" distance of L0.start A1.centre
  measures "d149" distance of L0.start A3.centre
  measures "d152" distance from line of L2 L0.start
  measures "d153" distance from line of L3 L0.start
extrude "Extrusion13" cut sketch "Sketch12" against normal blind 3 bodies 1
equation "\"d21\" = -0.5 * d15 + 0.5 * d20"
equation "\"d23\" = -0.5 * d18 + 0.5 * d22"
equation "\"d25\" = -0.5 * d24 + 0.5 * d14"
equation "\"d41\" = -0.5 * d39 + 0.5 * d40"
body "Solid1"
body "Solid2"
